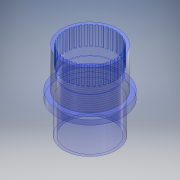
# Autodesk Inventor part: bague pour roue libre
Saved by Autodesk Inventor 2018.1 (Build 221171000, 171)
## iProperties
Created: 2022-05-09
Part Number: bague pour roue libre
Material: Generic
Document SubType Name: Modeling
Designer: Bureau
Density: 1 g/cm^3
Appearance: Default
Author: Bureau
Autodesk Inventor part; units mm, degrees
ref_plane "YZ Plane" through (0, 0, 0) normal (1, 0, 0) x (0, 1, 0)
ref_plane "XZ Plane" through (0, 0, 0) normal (0, 1, 0) x (-1, 0, 0)
ref_plane "XY Plane" through (0, 0, 0) normal (0, 0, 1) x (1, 0, 0)
sketch "Sketch1" plane through (0, 0, 0) normal (0, 0, 1) x (1, 0, 0)
  circle A0 centre (0, 0) radius 17.5
  circle A1 centre (0, 0) radius 12.5
  dimension "d0" = 35
  dimension "d1" = 25
  constraints: 2 centre point, 2 coincident
  measures "d0" diameter of A0
  measures "d1" diameter of A1
extrude "Extrusion1" add sketch "Sketch1" along normal blind 41.9
sketch "Sketch2" plane through (0, 0, 41.9) normal (0, 0, 1) x (1, 0, 0)
  circle A0 centre (0, 0) radius 13
  dimension "d4" = 26
  constraints: 1 centre point, 1 coincident
  measures "d4" diameter of A0
extrude "Extrusion2" cut sketch "Sketch2" against normal blind 14
sketch "Sketch3" plane through (0, 0, 41.9) normal (0, 0, 1) x (1, 0, 0)
  line L0 (0, 13) -> (1.02, 12.9599)
  line L1 (3.0348, 12.6408) -> (4.0172, 12.3637)
  line L2 (9.1924, 9.1924) -> (9.8853, 8.4428)
  line L3 (10.5172, 7.6412) -> (11.0843, 6.7925)
  line L4 (11.5831, 5.9019) -> (12.0104, 4.9749)
  line L5 (12.8399, 2.0336) -> (12.9599, 1.02)
  line L6 (13, 0) -> (12.9599, -1.02)
  line L7 (12.8399, -2.0336) -> (12.6408, -3.0348)
  line L8 (12.3637, -4.0172) -> (12.0104, -4.9749)
  line L9 (11.5831, -5.9019) -> (11.0843, -6.7925)
  line L10 (10.5172, -7.6412) -> (9.8853, -8.4428)
  line L11 (9.1924, -9.1924) -> (8.4428, -9.8853)
  line L12 (7.6412, -10.5172) -> (6.7925, -11.0843)
  line L13 (5.9019, -11.5831) -> (4.9749, -12.0104)
  line L14 (4.0172, -12.3637) -> (3.0348, -12.6408)
  line L15 (2.0336, -12.8399) -> (1.02, -12.9599)
  line L16 (-2.0336, -12.8399) -> (-3.0348, -12.6408)
  line L17 (-4.0172, -12.3637) -> (-4.9749, -12.0104)
  line L18 (-5.9019, -11.5831) -> (-6.7925, -11.0843)
  line L19 (-7.6412, -10.5172) -> (-8.4428, -9.8853)
  line L20 (-9.1924, -9.1924) -> (-9.8853, -8.4428)
  line L21 (-10.5172, -7.6412) -> (-11.0843, -6.7925)
  line L22 (-11.5831, -5.9019) -> (-12.0104, -4.9749)
  line L23 (-12.3637, -4.0172) -> (-12.6408, -3.0348)
  line L24 (-12.8399, -2.0336) -> (-12.9599, -1.02)
  line L25 (-13, 0) -> (-12.9599, 1.02)
  line L26 (-12.8399, 2.0336) -> (-12.6408, 3.0348)
  line L27 (-11.5831, 5.9019) -> (-11.0843, 6.7925)
  line L28 (-10.5172, 7.6412) -> (-9.8853, 8.4428)
  line L29 (-9.1924, 9.1924) -> (-8.4428, 9.8853)
  line L30 (-7.6412, 10.5172) -> (-6.7925, 11.0843)
  line L31 (-5.9019, 11.5831) -> (-4.9749, 12.0104)
  line L32 (-4.0172, 12.3637) -> (-3.0348, 12.6408)
  line L33 (0, 13) -> (0, 13.5)
  line L34 (1.02, 12.9599) -> (1.0592, 13.4584)
  arc A0 (1.0592, 13.4584) -> (0, 13.5) centre (0, 0) ccw
  arc A1 (-1.0592, 13.4584) -> (-2.1119, 13.3338) centre (0, 0) ccw
  line L35 (-1.02, 12.9599) -> (-1.0592, 13.4584)
  line L36 (-2.0336, 12.8399) -> (-1.02, 12.9599)
  line L37 (-2.0336, 12.8399) -> (-2.1119, 13.3338)
  arc A2 (-3.1515, 13.127) -> (-4.1717, 12.8393) centre (0, 0) ccw
  line L38 (-3.0348, 12.6408) -> (-3.1515, 13.127)
  line L39 (-4.0172, 12.3637) -> (-3.0348, 12.6408)
  line L40 (-4.0172, 12.3637) -> (-4.1717, 12.8393)
  arc A3 (-5.1662, 12.4724) -> (-6.1289, 12.0286) centre (0, 0) ccw
  line L41 (-4.9749, 12.0104) -> (-5.1662, 12.4724)
  line L42 (-5.9019, 11.5831) -> (-4.9749, 12.0104)
  line L43 (-5.9019, 11.5831) -> (-6.1289, 12.0286)
  arc A4 (-7.0537, 11.5106) -> (-7.9351, 10.9217) centre (0, 0) ccw
  line L44 (-6.7925, 11.0843) -> (-7.0537, 11.5106)
  line L45 (-7.6412, 10.5172) -> (-6.7925, 11.0843)
  line L46 (-7.6412, 10.5172) -> (-7.9351, 10.9217)
  arc A5 (-8.7675, 10.2655) -> (-9.5459, 9.5459) centre (0, 0) ccw
  line L47 (-8.4428, 9.8853) -> (-8.7675, 10.2655)
  line L48 (-9.1924, 9.1924) -> (-8.4428, 9.8853)
  line L49 (-9.1924, 9.1924) -> (-9.5459, 9.5459)
  arc A6 (-10.2655, 8.7675) -> (-10.9217, 7.9351) centre (0, 0) ccw
  line L50 (-9.8853, 8.4428) -> (-10.2655, 8.7675)
  line L51 (-10.5172, 7.6412) -> (-9.8853, 8.4428)
  line L52 (-10.5172, 7.6412) -> (-10.9217, 7.9351)
  arc A7 (-11.5106, 7.0537) -> (-12.0286, 6.1289) centre (0, 0) ccw
  line L53 (-11.0843, 6.7925) -> (-11.5106, 7.0537)
  line L54 (-11.5831, 5.9019) -> (-11.0843, 6.7925)
  line L55 (-11.5831, 5.9019) -> (-12.0286, 6.1289)
  arc A8 (-12.4724, 5.1662) -> (-12.8393, 4.1717) centre (0, 0) ccw
  line L56 (-12.0104, 4.9749) -> (-12.4724, 5.1662)
  line L57 (-12.3637, 4.0172) -> (-12.0104, 4.9749)
  line L58 (-12.3637, 4.0172) -> (-12.8393, 4.1717)
  arc A9 (-13.127, 3.1515) -> (-13.3338, 2.1119) centre (0, 0) ccw
  line L59 (-12.6408, 3.0348) -> (-13.127, 3.1515)
  line L60 (-12.8399, 2.0336) -> (-12.6408, 3.0348)
  line L61 (-12.8399, 2.0336) -> (-13.3338, 2.1119)
  arc A10 (-13.4584, 1.0592) -> (-13.5, 0) centre (0, 0) ccw
  line L62 (-12.9599, 1.02) -> (-13.4584, 1.0592)
  line L63 (-13, 0) -> (-12.9599, 1.02)
  line L64 (-13, 0) -> (-13.5, 0)
  arc A11 (-13.4584, -1.0592) -> (-13.3338, -2.1119) centre (0, 0) ccw
  line L65 (-12.9599, -1.02) -> (-13.4584, -1.0592)
  line L66 (-12.8399, -2.0336) -> (-12.9599, -1.02)
  line L67 (-12.8399, -2.0336) -> (-13.3338, -2.1119)
  arc A12 (-13.127, -3.1515) -> (-12.8393, -4.1717) centre (0, 0) ccw
  line L68 (-12.6408, -3.0348) -> (-13.127, -3.1515)
  line L69 (-12.3637, -4.0172) -> (-12.6408, -3.0348)
  line L70 (-12.3637, -4.0172) -> (-12.8393, -4.1717)
  arc A13 (-12.4724, -5.1662) -> (-12.0286, -6.1289) centre (0, 0) ccw
  line L71 (-12.0104, -4.9749) -> (-12.4724, -5.1662)
  line L72 (-11.5831, -5.9019) -> (-12.0104, -4.9749)
  line L73 (-11.5831, -5.9019) -> (-12.0286, -6.1289)
  arc A14 (-11.5106, -7.0537) -> (-10.9217, -7.9351) centre (0, 0) ccw
  line L74 (-11.0843, -6.7925) -> (-11.5106, -7.0537)
  line L75 (-10.5172, -7.6412) -> (-11.0843, -6.7925)
  line L76 (-10.5172, -7.6412) -> (-10.9217, -7.9351)
  arc A15 (-10.2655, -8.7675) -> (-9.5459, -9.5459) centre (0, 0) ccw
  line L77 (-9.8853, -8.4428) -> (-10.2655, -8.7675)
  line L78 (-9.1924, -9.1924) -> (-9.8853, -8.4428)
  line L79 (-9.1924, -9.1924) -> (-9.5459, -9.5459)
  arc A16 (-8.7675, -10.2655) -> (-7.9351, -10.9217) centre (0, 0) ccw
  line L80 (-8.4428, -9.8853) -> (-8.7675, -10.2655)
  line L81 (-7.6412, -10.5172) -> (-8.4428, -9.8853)
  line L82 (-7.6412, -10.5172) -> (-7.9351, -10.9217)
  arc A17 (-7.0537, -11.5106) -> (-6.1289, -12.0286) centre (0, 0) ccw
  line L83 (-6.7925, -11.0843) -> (-7.0537, -11.5106)
  line L84 (-5.9019, -11.5831) -> (-6.7925, -11.0843)
  line L85 (-5.9019, -11.5831) -> (-6.1289, -12.0286)
  arc A18 (-5.1662, -12.4724) -> (-4.1717, -12.8393) centre (0, 0) ccw
  line L86 (-4.9749, -12.0104) -> (-5.1662, -12.4724)
  line L87 (-4.0172, -12.3637) -> (-4.9749, -12.0104)
  line L88 (-4.0172, -12.3637) -> (-4.1717, -12.8393)
  arc A19 (-3.1515, -13.127) -> (-2.1119, -13.3338) centre (0, 0) ccw
  line L89 (-3.0348, -12.6408) -> (-3.1515, -13.127)
  line L90 (-2.0336, -12.8399) -> (-3.0348, -12.6408)
  line L91 (-2.0336, -12.8399) -> (-2.1119, -13.3338)
  arc A20 (-1.0592, -13.4584) -> (0, -13.5) centre (0, 0) ccw
  line L92 (-1.02, -12.9599) -> (-1.0592, -13.4584)
  line L93 (0, -13) -> (-1.02, -12.9599)
  line L94 (0, -13) -> (0, -13.5)
  arc A21 (1.0592, -13.4584) -> (2.1119, -13.3338) centre (0, 0) ccw
  line L95 (1.02, -12.9599) -> (1.0592, -13.4584)
  line L96 (2.0336, -12.8399) -> (1.02, -12.9599)
  line L97 (2.0336, -12.8399) -> (2.1119, -13.3338)
  arc A22 (3.1515, -13.127) -> (4.1717, -12.8393) centre (0, 0) ccw
  line L98 (3.0348, -12.6408) -> (3.1515, -13.127)
  line L99 (4.0172, -12.3637) -> (3.0348, -12.6408)
  line L100 (4.0172, -12.3637) -> (4.1717, -12.8393)
  arc A23 (5.1662, -12.4724) -> (6.1289, -12.0286) centre (0, 0) ccw
  line L101 (4.9749, -12.0104) -> (5.1662, -12.4724)
  line L102 (5.9019, -11.5831) -> (4.9749, -12.0104)
  line L103 (5.9019, -11.5831) -> (6.1289, -12.0286)
  arc A24 (7.0537, -11.5106) -> (7.9351, -10.9217) centre (0, 0) ccw
  line L104 (6.7925, -11.0843) -> (7.0537, -11.5106)
  line L105 (7.6412, -10.5172) -> (6.7925, -11.0843)
  line L106 (7.6412, -10.5172) -> (7.9351, -10.9217)
  arc A25 (8.7675, -10.2655) -> (9.5459, -9.5459) centre (0, 0) ccw
  line L107 (8.4428, -9.8853) -> (8.7675, -10.2655)
  line L108 (9.1924, -9.1924) -> (8.4428, -9.8853)
  line L109 (9.1924, -9.1924) -> (9.5459, -9.5459)
  arc A26 (10.2655, -8.7675) -> (10.9217, -7.9351) centre (0, 0) ccw
  line L110 (9.8853, -8.4428) -> (10.2655, -8.7675)
  line L111 (10.5172, -7.6412) -> (9.8853, -8.4428)
  line L112 (10.5172, -7.6412) -> (10.9217, -7.9351)
  arc A27 (11.5106, -7.0537) -> (12.0286, -6.1289) centre (0, 0) ccw
  line L113 (11.0843, -6.7925) -> (11.5106, -7.0537)
  line L114 (11.5831, -5.9019) -> (11.0843, -6.7925)
  line L115 (11.5831, -5.9019) -> (12.0286, -6.1289)
  arc A28 (12.4724, -5.1662) -> (12.8393, -4.1717) centre (0, 0) ccw
  line L116 (12.0104, -4.9749) -> (12.4724, -5.1662)
  line L117 (12.3637, -4.0172) -> (12.0104, -4.9749)
  line L118 (12.3637, -4.0172) -> (12.8393, -4.1717)
  arc A29 (13.127, -3.1515) -> (13.3338, -2.1119) centre (0, 0) ccw
  line L119 (12.6408, -3.0348) -> (13.127, -3.1515)
  line L120 (12.8399, -2.0336) -> (12.6408, -3.0348)
  line L121 (12.8399, -2.0336) -> (13.3338, -2.1119)
  arc A30 (13.4584, -1.0592) -> (13.5, 0) centre (0, 0) ccw
  line L122 (12.9599, -1.02) -> (13.4584, -1.0592)
  line L123 (13, 0) -> (12.9599, -1.02)
  line L124 (13, 0) -> (13.5, 0)
  arc A31 (13.4584, 1.0592) -> (13.3338, 2.1119) centre (0, 0) ccw
  line L125 (12.9599, 1.02) -> (13.4584, 1.0592)
  line L126 (12.8399, 2.0336) -> (12.9599, 1.02)
  line L127 (12.8399, 2.0336) -> (13.3338, 2.1119)
  arc A32 (13.127, 3.1515) -> (12.8393, 4.1717) centre (0, 0) ccw
  line L128 (12.6408, 3.0348) -> (13.127, 3.1515)
  line L129 (12.3637, 4.0172) -> (12.6408, 3.0348)
  line L130 (12.3637, 4.0172) -> (12.8393, 4.1717)
  arc A33 (12.4724, 5.1662) -> (12.0286, 6.1289) centre (0, 0) ccw
  line L131 (12.0104, 4.9749) -> (12.4724, 5.1662)
  line L132 (11.5831, 5.9019) -> (12.0104, 4.9749)
  line L133 (11.5831, 5.9019) -> (12.0286, 6.1289)
  arc A34 (11.5106, 7.0537) -> (10.9217, 7.9351) centre (0, 0) ccw
  line L134 (11.0843, 6.7925) -> (11.5106, 7.0537)
  line L135 (10.5172, 7.6412) -> (11.0843, 6.7925)
  line L136 (10.5172, 7.6412) -> (10.9217, 7.9351)
  arc A35 (10.2655, 8.7675) -> (9.5459, 9.5459) centre (0, 0) ccw
  line L137 (9.8853, 8.4428) -> (10.2655, 8.7675)
  line L138 (9.1924, 9.1924) -> (9.8853, 8.4428)
  line L139 (9.1924, 9.1924) -> (9.5459, 9.5459)
  arc A36 (8.7675, 10.2655) -> (7.9351, 10.9217) centre (0, 0) ccw
  line L140 (8.4428, 9.8853) -> (8.7675, 10.2655)
  line L141 (7.6412, 10.5172) -> (8.4428, 9.8853)
  line L142 (7.6412, 10.5172) -> (7.9351, 10.9217)
  arc A37 (7.0537, 11.5106) -> (6.1289, 12.0286) centre (0, 0) ccw
  line L143 (6.7925, 11.0843) -> (7.0537, 11.5106)
  line L144 (5.9019, 11.5831) -> (6.7925, 11.0843)
  line L145 (5.9019, 11.5831) -> (6.1289, 12.0286)
  arc A38 (5.1662, 12.4724) -> (4.1717, 12.8393) centre (0, 0) ccw
  line L146 (4.9749, 12.0104) -> (5.1662, 12.4724)
  line L147 (4.0172, 12.3637) -> (4.9749, 12.0104)
  line L148 (4.0172, 12.3637) -> (4.1717, 12.8393)
  arc A39 (3.1515, 13.127) -> (2.1119, 13.3338) centre (0, 0) ccw
  line L149 (3.0348, 12.6408) -> (3.1515, 13.127)
  line L150 (2.0336, 12.8399) -> (3.0348, 12.6408)
  line L151 (2.0336, 12.8399) -> (2.1119, 13.3338)
  point P0 (0, 0)
  point P1 (0, 0)
  point P2 (0, 0)
  dimension "d9" = 27
  dimension "d12" = 360
  constraints: 304 end point, 80 point on circle, 40 centre point, 1 vertical, 422 other
  measures "d9" diameter of A0
extrude "Extrusion3" cut sketch "Sketch3" against normal blind 10
sketch "Sketch5" plane through (0, 0, 41.9) normal (0, 0, 1) x (1, 0, 0)
  circle A0 centre (0, 0) radius 15
  circle A1 centre (0, 0) radius 17.5
  dimension "d31" = 30
  dimension "d32" = 35
  constraints: 2 centre point, 2 coincident
  measures "d31" diameter of A0
  measures "d32" diameter of A1
extrude "Extrusion4" cut sketch "Sketch5" against normal blind 21
thread "Thread1" size "M30x1" class "6g" standard "ANSI Metric M Profile" full length
sketch "Sketch6" plane through (0, 0, 0) normal (0, 0, -1) x (-1, 0, 0)
  circle A0 centre (0, 0) radius 14
  circle A1 centre (0, 0) radius 17.5
  dimension "d37" = 28
  dimension "d38" = 35
  constraints: 2 centre point, 2 coincident
  measures "d37" diameter of A0
  measures "d38" diameter of A1
extrude "Extrusion5" cut sketch "Sketch6" against normal blind 17
body "Solid1"
